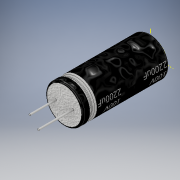
# Autodesk Inventor part: capacitor 2
Saved by Autodesk Inventor 2019 (Build 230136000, 136)
## iProperties
Created: 2019-08-10
Part Number: capacitor 2
Material: Типовые
Document SubType Name: Modeling
Designer: azizg
Density: 1 g/cm^3
Appearance: По умолчанию
Author: azizg
Autodesk Inventor part; units mm, degrees
sketch "Эскиз1" plane through (0, 0, 0) normal (0, 0, 1) x (1, 0, 0)
  line L0 (-13.3395, 0) -> (13.3395, 0)
  line L1 (0, 13.3395) -> (0, -13.3395)
  circle A0 centre (0, 0) radius 11
  dimension "d0" = 22
  constraints: 6 midpoint, 4 end point, 1 centre point, 1 coincident, 1 horizontal, 1 vertical
  measures "d0" diameter of A0
extrude "Выдавливание1" add sketch "Эскиз1" along normal mid plane 50
ref_plane "РабПлоскость3" through (0, 0, 20) normal (0, 0, 1) x (1, 0, 0)
sketch "Эскиз3" plane through (0, 0, 20) normal (0, 0, 1) x (1, 0, 0)
  line L0 (-22, 0) -> (25.1429, 0)
  line L1 (0, 25.1429) -> (0, -23.5714)
  circle A0 centre (0, 0) radius 11
  circle A1 centre (0, 0) radius 10
  dimension "d5" = 22
  dimension "d6" = 20
  constraints: 4 end point, 2 centre point, 2 coincident, 2 point on line, 1 horizontal, 1 vertical
  measures "d5" diameter of A0
  measures "d6" diameter of A1
extrude "Выдавливание2" cut sketch "Эскиз3" against normal blind 2 contours A1 L1 A0 L0 | L0 A0 L1 A1 | A1 L0 A0 L1 | L1 A0 L0 A1
fillet "Сопряжение1" radius 1 6 edges at (-11, 0, 20) (-11, 0, 18) (-10, 0, 18) (-10, 0, 20) (-11, 0, 25) (-11, 0, -25)
sketch "Эскиз4" plane through (0, 0, -25) normal (0, 0, -1) x (-1, 0, 0)
  line L0 (1.547, 4.223) -> (-2.9486, 4.223) construction
  line L1 (-2.9486, 4.223) -> (-2.9486, -4.5142) construction
  line L2 (-2.9486, -4.5142) -> (1.547, -4.5142) construction
  line L3 (1.547, -4.5142) -> (1.547, 4.223) construction
  line L4 (-1.1823, 0.0186) -> (-0.1499, 0.0186)
  line L5 (-0.1499, 0.0186) -> (-0.1499, 1.0511)
  line L6 (-0.1499, 1.0511) -> (0.191, 1.0511)
  line L7 (0.191, 1.0511) -> (0.191, 0.0186)
  line L8 (0.191, 0.0186) -> (1.2235, 0.0186)
  line L9 (1.2235, 0.0186) -> (1.2235, -0.3099)
  line L10 (1.2235, -0.3099) -> (0.191, -0.3099)
  line L11 (0.191, -0.3099) -> (0.191, -1.3423)
  line L12 (0.191, -1.3423) -> (-0.1499, -1.3423)
  line L13 (-0.1499, -1.3423) -> (-0.1499, -0.3099)
  line L14 (-0.1499, -0.3099) -> (-1.1823, -0.3099)
  line L15 (-1.1823, -0.3099) -> (-1.1823, 0.0186)
  point P0 (0, 0)
  dimension "d0" = 22
  constraints: 2 other
extrude "Выдавливание3" add sketch "Эскиз4" against normal blind 0.1
sketch "Эскиз5" plane through (0, 0, -25) normal (0, 0, -1) x (-1, 0, 0)
  line L0 (-1.5437, 1.0709) -> (1.5067, 1.0709) construction
  line L1 (1.5067, 1.0709) -> (1.5067, -1.3226) construction
  line L2 (1.5067, -1.3226) -> (-1.5437, -1.3226) construction
  line L3 (-1.5437, -1.3226) -> (-1.5437, 1.0709) construction
  line L4 (1.1856, -0.2901) -> (0.1532, -0.2901)
  line L5 (0.1532, -0.2901) -> (0.1532, -1.3226)
  line L6 (0.1532, -1.3226) -> (-0.1877, -1.3226)
  line L7 (-0.1877, -1.3226) -> (-0.1877, -0.2901)
  line L8 (-0.1877, -0.2901) -> (-1.2202, -0.2901)
  line L9 (-1.2202, -0.2901) -> (-1.2202, 0.0384)
  line L10 (-1.2202, 0.0384) -> (-0.1877, 0.0384)
  line L11 (-0.1877, 0.0384) -> (-0.1877, 1.0709)
  line L12 (-0.1877, 1.0709) -> (0.1532, 1.0709)
  line L13 (0.1532, 1.0709) -> (0.1532, 0.0384)
  line L14 (0.1532, 0.0384) -> (1.1856, 0.0384)
  line L15 (1.1856, 0.0384) -> (1.1856, -0.2901)
  point P0 (0, 0)
  dimension "d0" = 22
  constraints: 2 other
extrude "Выдавливание4" add sketch "Эскиз5" against normal blind 0.1
ref_plane "РабПлоскость4" through (11, 0, 0) normal (1, 0, 0) x (0, 1, 0)
sketch "Эскиз6" plane through (11, 0, 0) normal (1, 0, 0) x (0, 1, 0)
  line L0 (-4.859, -23.88) -> (-4.859, -8.4004) construction
  line L1 (-4.859, -8.4004) -> (3.8671, -8.4004) construction
  line L2 (3.8671, -8.4004) -> (3.8671, -23.88) construction
  line L3 (3.8671, -23.88) -> (-4.859, -23.88) construction
  line L4 (-5.3548, 2.6762) -> (-5.3548, 16.9441) construction
  line L5 (-5.3548, 16.9441) -> (3.3351, 16.9441) construction
  line L6 (3.3351, 16.9441) -> (3.3351, 2.6762) construction
  line L7 (3.3351, 2.6762) -> (-5.3548, 2.6762) construction
  line L8 (-1.7493, -21.9312) -> (-1.7493, -23.4181)
  line L9 (-1.7493, -23.4181) -> (-2.0605, -23.4181)
  line L10 (-2.0605, -23.4181) -> (-2.0605, -22.8648)
  line L11 (-2.0605, -22.8648) -> (-4.1032, -22.8648)
  line L12 (-4.1032, -22.8648) -> (-4.1032, -23.4181)
  line L13 (-4.1032, -23.4181) -> (-4.3823, -23.4181)
  spline S0 degree 2 poles (-4.3823, -23.4181) (-4.3823, -23.1044) (-4.5601, -22.808) (-4.8071, -22.7883) knots 0 0 0 1 2 2 2
  line L14 (-4.8071, -22.7883) -> (-4.8071, -22.4721)
  line L15 (-4.8071, -22.4721) -> (-2.0605, -22.4721)
  line L16 (-2.0605, -22.4721) -> (-2.0605, -21.9312)
  line L17 (-2.0605, -21.9312) -> (-1.7493, -21.9312)
  spline S1 degree 2 poles (-3.2733, -19.4735) (-2.4532, -19.4735) (-1.685, -19.9502) (-1.685, -20.4467) knots 0 0 0 1 2 2 2
  spline S2 degree 2 poles (-1.685, -20.4467) (-1.685, -20.9506) (-2.468, -21.4223) (-3.2708, -21.4223) knots 0 0 0 1 2 2 2
  spline S3 degree 2 poles (-3.2708, -21.4223) (-4.0958, -21.4223) (-4.859, -20.9456) (-4.859, -20.4467) knots 0 0 0 1 2 2 2
  spline S4 degree 2 poles (-4.859, -20.4467) (-4.859, -19.9453) (-4.0686, -19.4735) (-3.2733, -19.4735) knots 0 0 0 1 2 2 2
  spline S5 degree 2 poles (-2.3445, -19.9971) (-2.4952, -19.9379) (-2.9596, -19.8885) (-3.2733, -19.8885) knots 0 0 0 1 2 2 2
  spline S6 degree 2 poles (-3.2733, -19.8885) (-3.5869, -19.8885) (-4.0488, -19.9379) (-4.2044, -19.9996) knots 0 0 0 1 2 2 2
  spline S7 degree 2 poles (-4.2044, -19.9996) (-4.3601, -20.0614) (-4.5206, -20.2763) (-4.5206, -20.4467) knots 0 0 0 1 2 2 2
  spline S8 degree 2 poles (-4.5206, -20.4467) (-4.5206, -20.6171) (-4.3601, -20.8369) (-4.1995, -20.9012) knots 0 0 0 1 2 2 2
  spline S9 degree 2 poles (-4.1995, -20.9012) (-4.0439, -20.9629) (-3.5697, -21.0074) (-3.2708, -21.0074) knots 0 0 0 1 2 2 2
  spline S10 degree 2 poles (-3.2708, -21.0074) (-2.9497, -21.0074) (-2.5199, -20.9679) (-2.3519, -20.9036) knots 0 0 0 1 2 2 2
  spline S11 degree 2 poles (-2.3519, -20.9036) (-2.1939, -20.8444) (-2.0234, -20.6245) (-2.0234, -20.4467) knots 0 0 0 1 2 2 2
  spline S12 degree 2 poles (-2.0234, -20.4467) (-2.0234, -20.2787) (-2.184, -20.0589) (-2.3445, -19.9971) knots 0 0 0 1 2 2 2
  spline S13 degree 2 poles (-3.2733, -17.1863) (-2.4532, -17.1863) (-1.685, -17.663) (-1.685, -18.1594) knots 0 0 0 1 2 2 2
  spline S14 degree 2 poles (-1.685, -18.1594) (-1.685, -18.6633) (-2.468, -19.1351) (-3.2708, -19.1351) knots 0 0 0 1 2 2 2
  spline S15 degree 2 poles (-3.2708, -19.1351) (-4.0958, -19.1351) (-4.859, -18.6584) (-4.859, -18.1594) knots 0 0 0 1 2 2 2
  spline S16 degree 2 poles (-4.859, -18.1594) (-4.859, -17.658) (-4.0686, -17.1863) (-3.2733, -17.1863) knots 0 0 0 1 2 2 2
  spline S17 degree 2 poles (-2.3445, -17.7099) (-2.4952, -17.6506) (-2.9596, -17.6012) (-3.2733, -17.6012) knots 0 0 0 1 2 2 2
  spline S18 degree 2 poles (-3.2733, -17.6012) (-3.5869, -17.6012) (-4.0488, -17.6506) (-4.2044, -17.7124) knots 0 0 0 1 2 2 2
  spline S19 degree 2 poles (-4.2044, -17.7124) (-4.3601, -17.7741) (-4.5206, -17.989) (-4.5206, -18.1594) knots 0 0 0 1 2 2 2
  spline S20 degree 2 poles (-4.5206, -18.1594) (-4.5206, -18.3299) (-4.3601, -18.5497) (-4.1995, -18.6139) knots 0 0 0 1 2 2 2
  spline S21 degree 2 poles (-4.1995, -18.6139) (-4.0439, -18.6757) (-3.5697, -18.7201) (-3.2708, -18.7201) knots 0 0 0 1 2 2 2
  spline S22 degree 2 poles (-3.2708, -18.7201) (-2.9497, -18.7201) (-2.5199, -18.6806) (-2.3519, -18.6164) knots 0 0 0 1 2 2 2
  spline S23 degree 2 poles (-2.3519, -18.6164) (-2.1939, -18.5571) (-2.0234, -18.3373) (-2.0234, -18.1594) knots 0 0 0 1 2 2 2
  spline S24 degree 2 poles (-2.0234, -18.1594) (-2.0234, -17.9915) (-2.184, -17.7717) (-2.3445, -17.7099) knots 0 0 0 1 2 2 2
  line L18 (-4.7973, -14.4989) -> (-1.7493, -15.5486)
  line L19 (-1.7493, -15.5486) -> (-1.7493, -15.9858)
  line L20 (-1.7493, -15.9858) -> (-4.7973, -17.0356)
  line L21 (-4.7973, -17.0356) -> (-4.7973, -16.6009)
  line L22 (-4.7973, -16.6009) -> (-2.2655, -15.7561)
  line L23 (-2.2655, -15.7561) -> (-4.7973, -14.9114)
  line L24 (-4.7973, -14.9114) -> (-4.7973, -14.4989)
  line L25 (3.2692, -21.778) -> (3.2692, -23.6577)
  line L26 (3.2692, -23.6577) -> (2.8369, -23.6577)
  spline S25 degree 2 poles (2.8369, -23.6577) (2.6468, -23.4552) (2.2935, -23.0945) (2.1034, -22.9216) knots 0 0 0 1 2 2 2
  spline S26 degree 2 poles (2.1034, -22.9216) (1.7205, -22.5734) (1.2611, -22.319) (1.0165, -22.319) knots 0 0 0 1 2 2 2
  spline S27 degree 2 poles (1.0165, -22.319) (0.8881, -22.319) (0.6954, -22.398) (0.6337, -22.4696) knots 0 0 0 1 2 2 2
  spline S28 degree 2 poles (0.6337, -22.4696) (0.5719, -22.5413) (0.5102, -22.729) (0.5102, -22.8426) knots 0 0 0 1 2 2 2
  spline S29 degree 2 poles (0.5102, -22.8426) (0.5102, -22.9513) (0.5645, -23.1736) (0.6065, -23.2749) knots 0 0 0 1 2 2 2
  spline S30 degree 2 poles (0.6065, -23.2749) (0.6411, -23.3613) (0.7399, -23.5219) (0.7745, -23.5713) knots 0 0 0 1 2 2 2
  line L27 (0.7745, -23.5713) -> (0.7745, -23.5935)
  line L28 (0.7745, -23.5935) -> (0.3398, -23.5935)
  spline S31 degree 2 poles (0.3398, -23.5935) (0.278, -23.4675) (0.157, -23.0155) (0.157, -22.813) knots 0 0 0 1 2 2 2
  spline S32 degree 2 poles (0.157, -22.813) (0.157, -22.3856) (0.609, -21.904) (0.9943, -21.904) knots 0 0 0 1 2 2 2
  spline S33 degree 2 poles (0.9943, -21.904) (1.1746, -21.904) (1.476, -21.988) (1.6044, -22.0621) knots 0 0 0 1 2 2 2
  spline S34 degree 2 poles (1.6044, -22.0621) (1.7378, -22.1362) (1.9996, -22.3511) (2.1256, -22.4696) knots 0 0 0 1 2 2 2
  spline S35 degree 2 poles (2.1256, -22.4696) (2.3355, -22.6623) (2.7851, -23.1341) (2.916, -23.2749) knots 0 0 0 1 2 2 2
  line L29 (2.916, -23.2749) -> (2.916, -21.778)
  line L30 (2.916, -21.778) -> (3.2692, -21.778)
  line L31 (3.2692, -19.4908) -> (3.2692, -21.3705)
  line L32 (3.2692, -21.3705) -> (2.8369, -21.3705)
  spline S36 degree 2 poles (2.8369, -21.3705) (2.6468, -21.1679) (2.2935, -20.8073) (2.1034, -20.6344) knots 0 0 0 1 2 2 2
  spline S37 degree 2 poles (2.1034, -20.6344) (1.7205, -20.2861) (1.2611, -20.0317) (1.0165, -20.0317) knots 0 0 0 1 2 2 2
  spline S38 degree 2 poles (1.0165, -20.0317) (0.8881, -20.0317) (0.6954, -20.1108) (0.6337, -20.1824) knots 0 0 0 1 2 2 2
  spline S39 degree 2 poles (0.6337, -20.1824) (0.5719, -20.254) (0.5102, -20.4417) (0.5102, -20.5554) knots 0 0 0 1 2 2 2
  spline S40 degree 2 poles (0.5102, -20.5554) (0.5102, -20.664) (0.5645, -20.8863) (0.6065, -20.9876) knots 0 0 0 1 2 2 2
  spline S41 degree 2 poles (0.6065, -20.9876) (0.6411, -21.0741) (0.7399, -21.2346) (0.7745, -21.284) knots 0 0 0 1 2 2 2
  line L33 (0.7745, -21.284) -> (0.7745, -21.3063)
  line L34 (0.7745, -21.3063) -> (0.3398, -21.3063)
  spline S42 degree 2 poles (0.3398, -21.3063) (0.278, -21.1803) (0.157, -20.7283) (0.157, -20.5257) knots 0 0 0 1 2 2 2
  spline S43 degree 2 poles (0.157, -20.5257) (0.157, -20.0984) (0.609, -19.6168) (0.9943, -19.6168) knots 0 0 0 1 2 2 2
  spline S44 degree 2 poles (0.9943, -19.6168) (1.1746, -19.6168) (1.476, -19.7007) (1.6044, -19.7748) knots 0 0 0 1 2 2 2
  spline S45 degree 2 poles (1.6044, -19.7748) (1.7378, -19.8489) (1.9996, -20.0638) (2.1256, -20.1824) knots 0 0 0 1 2 2 2
  spline S46 degree 2 poles (2.1256, -20.1824) (2.3355, -20.3751) (2.7851, -20.8468) (2.916, -20.9876) knots 0 0 0 1 2 2 2
  line L35 (2.916, -20.9876) -> (2.916, -19.4908)
  line L36 (2.916, -19.4908) -> (3.2692, -19.4908)
  spline S47 degree 2 poles (1.7452, -17.1863) (2.5652, -17.1863) (3.3334, -17.663) (3.3334, -18.1594) knots 0 0 0 1 2 2 2
  spline S48 degree 2 poles (3.3334, -18.1594) (3.3334, -18.6633) (2.5504, -19.1351) (1.7477, -19.1351) knots 0 0 0 1 2 2 2
  spline S49 degree 2 poles (1.7477, -19.1351) (0.9227, -19.1351) (0.1595, -18.6584) (0.1595, -18.1594) knots 0 0 0 1 2 2 2
  spline S50 degree 2 poles (0.1595, -18.1594) (0.1595, -17.658) (0.9499, -17.1863) (1.7452, -17.1863) knots 0 0 0 1 2 2 2
  spline S51 degree 2 poles (2.6739, -17.7099) (2.5233, -17.6506) (2.0589, -17.6012) (1.7452, -17.6012) knots 0 0 0 1 2 2 2
  spline S52 degree 2 poles (1.7452, -17.6012) (1.4315, -17.6012) (0.9696, -17.6506) (0.814, -17.7124) knots 0 0 0 1 2 2 2
  spline S53 degree 2 poles (0.814, -17.7124) (0.6584, -17.7741) (0.4978, -17.989) (0.4978, -18.1594) knots 0 0 0 1 2 2 2
  spline S54 degree 2 poles (0.4978, -18.1594) (0.4978, -18.3299) (0.6584, -18.5497) (0.8189, -18.6139) knots 0 0 0 1 2 2 2
  spline S55 degree 2 poles (0.8189, -18.6139) (0.9746, -18.6757) (1.4488, -18.7201) (1.7477, -18.7201) knots 0 0 0 1 2 2 2
  spline S56 degree 2 poles (1.7477, -18.7201) (2.0688, -18.7201) (2.4986, -18.6806) (2.6665, -18.6164) knots 0 0 0 1 2 2 2
  spline S57 degree 2 poles (2.6665, -18.6164) (2.8246, -18.5571) (2.995, -18.3373) (2.995, -18.1594) knots 0 0 0 1 2 2 2
  spline S58 degree 2 poles (2.995, -18.1594) (2.995, -17.9915) (2.8345, -17.7717) (2.6739, -17.7099) knots 0 0 0 1 2 2 2
  spline S59 degree 2 poles (1.7452, -14.899) (2.5652, -14.899) (3.3334, -15.3757) (3.3334, -15.8722) knots 0 0 0 1 2 2 2
  spline S60 degree 2 poles (3.3334, -15.8722) (3.3334, -16.3761) (2.5504, -16.8479) (1.7477, -16.8479) knots 0 0 0 1 2 2 2
  spline S61 degree 2 poles (1.7477, -16.8479) (0.9227, -16.8479) (0.1595, -16.3712) (0.1595, -15.8722) knots 0 0 0 1 2 2 2
  spline S62 degree 2 poles (0.1595, -15.8722) (0.1595, -15.3708) (0.9499, -14.899) (1.7452, -14.899) knots 0 0 0 1 2 2 2
  spline S63 degree 2 poles (2.6739, -15.4227) (2.5233, -15.3634) (2.0589, -15.314) (1.7452, -15.314) knots 0 0 0 1 2 2 2
  spline S64 degree 2 poles (1.7452, -15.314) (1.4315, -15.314) (0.9696, -15.3634) (0.814, -15.4251) knots 0 0 0 1 2 2 2
  spline S65 degree 2 poles (0.814, -15.4251) (0.6584, -15.4869) (0.4978, -15.7018) (0.4978, -15.8722) knots 0 0 0 1 2 2 2
  spline S66 degree 2 poles (0.4978, -15.8722) (0.4978, -16.0426) (0.6584, -16.2625) (0.8189, -16.3267) knots 0 0 0 1 2 2 2
  spline S67 degree 2 poles (0.8189, -16.3267) (0.9746, -16.3884) (1.4488, -16.4329) (1.7477, -16.4329) knots 0 0 0 1 2 2 2
  spline S68 degree 2 poles (1.7477, -16.4329) (2.0688, -16.4329) (2.4986, -16.3934) (2.6665, -16.3292) knots 0 0 0 1 2 2 2
  spline S69 degree 2 poles (2.6665, -16.3292) (2.8246, -16.2699) (2.995, -16.0501) (2.995, -15.8722) knots 0 0 0 1 2 2 2
  spline S70 degree 2 poles (2.995, -15.8722) (2.995, -15.7043) (2.8345, -15.4844) (2.6739, -15.4227) knots 0 0 0 1 2 2 2
  line L37 (3.2692, -12.6735) -> (3.2692, -13.0589)
  line L38 (3.2692, -13.0589) -> (3.0173, -13.0589)
  spline S71 degree 2 poles (3.0173, -13.0589) (3.1729, -13.2367) (3.3334, -13.5553) (3.3334, -13.7529) knots 0 0 0 1 2 2 2
  spline S72 degree 2 poles (3.3334, -13.7529) (3.3334, -13.9011) (3.2346, -14.1654) (3.1284, -14.2618) knots 0 0 0 1 2 2 2
  spline S73 degree 2 poles (3.1284, -14.2618) (3.0222, -14.3606) (2.6986, -14.4692) (2.4664, -14.4692) knots 0 0 0 1 2 2 2
  line L39 (2.4664, -14.4692) -> (0.982, -14.4692)
  line L40 (0.982, -14.4692) -> (0.982, -14.0839)
  line L41 (0.982, -14.0839) -> (2.2861, -14.0839)
  spline S74 degree 2 poles (2.2861, -14.0839) (2.4689, -14.0839) (2.7085, -14.0568) (2.7974, -14.0098) knots 0 0 0 1 2 2 2
  spline S75 degree 2 poles (2.7974, -14.0098) (2.8863, -13.9629) (2.9679, -13.8023) (2.9679, -13.6517) knots 0 0 0 1 2 2 2
  spline S76 degree 2 poles (2.9679, -13.6517) (2.9679, -13.5109) (2.8073, -13.1922) (2.6912, -13.0589) knots 0 0 0 1 2 2 2
  line L42 (2.6912, -13.0589) -> (0.982, -13.0589)
  line L43 (0.982, -13.0589) -> (0.982, -12.6735)
  line L44 (0.982, -12.6735) -> (3.2692, -12.6735)
  line L45 (0.5818, -10.2628) -> (0.5818, -11.6806)
  line L46 (0.5818, -11.6806) -> (1.4414, -11.6806)
  line L47 (1.4414, -11.6806) -> (1.4414, -10.3221)
  line L48 (1.4414, -10.3221) -> (1.802, -10.3221)
  line L49 (1.802, -10.3221) -> (1.802, -11.6806)
  line L50 (1.802, -11.6806) -> (3.2692, -11.6806)
  line L51 (3.2692, -11.6806) -> (3.2692, -12.0857)
  line L52 (3.2692, -12.0857) -> (0.2212, -12.0857)
  line L53 (0.2212, -12.0857) -> (0.2212, -10.2628)
  line L54 (0.2212, -10.2628) -> (0.5818, -10.2628)
  line L55 (-2.245, 4.6251) -> (-2.245, 3.1381)
  line L56 (-2.245, 3.1381) -> (-2.5562, 3.1381)
  line L57 (-2.5562, 3.1381) -> (-2.5562, 3.6914)
  line L58 (-2.5562, 3.6914) -> (-4.5989, 3.6914)
  line L59 (-4.5989, 3.6914) -> (-4.5989, 3.1381)
  line L60 (-4.5989, 3.1381) -> (-4.878, 3.1381)
  spline S77 degree 2 poles (-4.878, 3.1381) (-4.878, 3.4518) (-5.0559, 3.7482) (-5.3029, 3.768) knots 0 0 0 1 2 2 2
  line L61 (-5.3029, 3.768) -> (-5.3029, 4.0841)
  line L62 (-5.3029, 4.0841) -> (-2.5562, 4.0841)
  line L63 (-2.5562, 4.0841) -> (-2.5562, 4.6251)
  line L64 (-2.5562, 4.6251) -> (-2.245, 4.6251)
  spline S78 degree 2 poles (-3.769, 7.0827) (-2.949, 7.0827) (-2.1808, 6.606) (-2.1808, 6.1095) knots 0 0 0 1 2 2 2
  spline S79 degree 2 poles (-2.1808, 6.1095) (-2.1808, 5.6057) (-2.9638, 5.1339) (-3.7665, 5.1339) knots 0 0 0 1 2 2 2
  spline S80 degree 2 poles (-3.7665, 5.1339) (-4.5915, 5.1339) (-5.3548, 5.6106) (-5.3548, 6.1095) knots 0 0 0 1 2 2 2
  spline S81 degree 2 poles (-5.3548, 6.1095) (-5.3548, 6.611) (-4.5643, 7.0827) (-3.769, 7.0827) knots 0 0 0 1 2 2 2
  spline S82 degree 2 poles (-2.8403, 6.5591) (-2.9909, 6.6184) (-3.4553, 6.6678) (-3.769, 6.6678) knots 0 0 0 1 2 2 2
  spline S83 degree 2 poles (-3.769, 6.6678) (-4.0827, 6.6678) (-4.5446, 6.6184) (-4.7002, 6.5566) knots 0 0 0 1 2 2 2
  spline S84 degree 2 poles (-4.7002, 6.5566) (-4.8558, 6.4949) (-5.0164, 6.28) (-5.0164, 6.1095) knots 0 0 0 1 2 2 2
  spline S85 degree 2 poles (-5.0164, 6.1095) (-5.0164, 5.9391) (-4.8558, 5.7193) (-4.6953, 5.6551) knots 0 0 0 1 2 2 2
  spline S86 degree 2 poles (-4.6953, 5.6551) (-4.5396, 5.5933) (-4.0654, 5.5488) (-3.7665, 5.5488) knots 0 0 0 1 2 2 2
  spline S87 degree 2 poles (-3.7665, 5.5488) (-3.4454, 5.5488) (-3.0156, 5.5884) (-2.8477, 5.6526) knots 0 0 0 1 2 2 2
  spline S88 degree 2 poles (-2.8477, 5.6526) (-2.6896, 5.7119) (-2.5192, 5.9317) (-2.5192, 6.1095) knots 0 0 0 1 2 2 2
  spline S89 degree 2 poles (-2.5192, 6.1095) (-2.5192, 6.2775) (-2.6797, 6.4973) (-2.8403, 6.5591) knots 0 0 0 1 2 2 2
  spline S90 degree 2 poles (-3.769, 9.37) (-2.949, 9.37) (-2.1808, 8.8932) (-2.1808, 8.3968) knots 0 0 0 1 2 2 2
  spline S91 degree 2 poles (-2.1808, 8.3968) (-2.1808, 7.8929) (-2.9638, 7.4211) (-3.7665, 7.4211) knots 0 0 0 1 2 2 2
  spline S92 degree 2 poles (-3.7665, 7.4211) (-4.5915, 7.4211) (-5.3548, 7.8978) (-5.3548, 8.3968) knots 0 0 0 1 2 2 2
  spline S93 degree 2 poles (-5.3548, 8.3968) (-5.3548, 8.8982) (-4.5643, 9.37) (-3.769, 9.37) knots 0 0 0 1 2 2 2
  spline S94 degree 2 poles (-2.8403, 8.8463) (-2.9909, 8.9056) (-3.4553, 8.955) (-3.769, 8.955) knots 0 0 0 1 2 2 2
  spline S95 degree 2 poles (-3.769, 8.955) (-4.0827, 8.955) (-4.5446, 8.9056) (-4.7002, 8.8438) knots 0 0 0 1 2 2 2
  spline S96 degree 2 poles (-4.7002, 8.8438) (-4.8558, 8.7821) (-5.0164, 8.5672) (-5.0164, 8.3968) knots 0 0 0 1 2 2 2
  spline S97 degree 2 poles (-5.0164, 8.3968) (-5.0164, 8.2263) (-4.8558, 8.0065) (-4.6953, 7.9423) knots 0 0 0 1 2 2 2
  spline S98 degree 2 poles (-4.6953, 7.9423) (-4.5396, 7.8805) (-4.0654, 7.8361) (-3.7665, 7.8361) knots 0 0 0 1 2 2 2
  spline S99 degree 2 poles (-3.7665, 7.8361) (-3.4454, 7.8361) (-3.0156, 7.8756) (-2.8477, 7.9398) knots 0 0 0 1 2 2 2
  spline S100 degree 2 poles (-2.8477, 7.9398) (-2.6896, 7.9991) (-2.5192, 8.2189) (-2.5192, 8.3968) knots 0 0 0 1 2 2 2
  spline S101 degree 2 poles (-2.5192, 8.3968) (-2.5192, 8.5647) (-2.6797, 8.7846) (-2.8403, 8.8463) knots 0 0 0 1 2 2 2
  line L65 (-5.293, 12.0573) -> (-2.245, 11.0076)
  line L66 (-2.245, 11.0076) -> (-2.245, 10.5704)
  line L67 (-2.245, 10.5704) -> (-5.293, 9.5206)
  line L68 (-5.293, 9.5206) -> (-5.293, 9.9554)
  line L69 (-5.293, 9.9554) -> (-2.7612, 10.8001)
  line L70 (-2.7612, 10.8001) -> (-5.293, 11.6448)
  line L71 (-5.293, 11.6448) -> (-5.293, 12.0573)
  line L72 (2.7735, 4.7782) -> (2.7735, 2.8985)
  line L73 (2.7735, 2.8985) -> (2.3412, 2.8985)
  spline S102 degree 2 poles (2.3412, 2.8985) (2.151, 3.1011) (1.7978, 3.4617) (1.6076, 3.6346) knots 0 0 0 1 2 2 2
  spline S103 degree 2 poles (1.6076, 3.6346) (1.2248, 3.9829) (0.7653, 4.2373) (0.5208, 4.2373) knots 0 0 0 1 2 2 2
  spline S104 degree 2 poles (0.5208, 4.2373) (0.3924, 4.2373) (0.1997, 4.1582) (0.1379, 4.0866) knots 0 0 0 1 2 2 2
  spline S105 degree 2 poles (0.1379, 4.0866) (0.0762, 4.015) (0.0144, 3.8272) (0.0144, 3.7136) knots 0 0 0 1 2 2 2
  spline S106 degree 2 poles (0.0144, 3.7136) (0.0144, 3.6049) (0.0688, 3.3826) (0.1108, 3.2814) knots 0 0 0 1 2 2 2
  spline S107 degree 2 poles (0.1108, 3.2814) (0.1454, 3.1949) (0.2442, 3.0344) (0.2787, 2.985) knots 0 0 0 1 2 2 2
  line L74 (0.2787, 2.985) -> (0.2787, 2.9627)
  line L75 (0.2787, 2.9627) -> (-0.156, 2.9627)
  spline S108 degree 2 poles (-0.156, 2.9627) (-0.2177, 3.0887) (-0.3388, 3.5407) (-0.3388, 3.7433) knots 0 0 0 1 2 2 2
  spline S109 degree 2 poles (-0.3388, 3.7433) (-0.3388, 4.1706) (0.1132, 4.6522) (0.4986, 4.6522) knots 0 0 0 1 2 2 2
  spline S110 degree 2 poles (0.4986, 4.6522) (0.6789, 4.6522) (0.9802, 4.5682) (1.1087, 4.4941) knots 0 0 0 1 2 2 2
  spline S111 degree 2 poles (1.1087, 4.4941) (1.242, 4.42) (1.5039, 4.2052) (1.6298, 4.0866) knots 0 0 0 1 2 2 2
  spline S112 degree 2 poles (1.6298, 4.0866) (1.8398, 3.8939) (2.2893, 3.4222) (2.4202, 3.2814) knots 0 0 0 1 2 2 2
  line L76 (2.4202, 3.2814) -> (2.4202, 4.7782)
  line L77 (2.4202, 4.7782) -> (2.7735, 4.7782)
  line L78 (2.7735, 7.0654) -> (2.7735, 5.1858)
  line L79 (2.7735, 5.1858) -> (2.3412, 5.1858)
  spline S113 degree 2 poles (2.3412, 5.1858) (2.151, 5.3883) (1.7978, 5.7489) (1.6076, 5.9218) knots 0 0 0 1 2 2 2
  spline S114 degree 2 poles (1.6076, 5.9218) (1.2248, 6.2701) (0.7653, 6.5245) (0.5208, 6.5245) knots 0 0 0 1 2 2 2
  spline S115 degree 2 poles (0.5208, 6.5245) (0.3924, 6.5245) (0.1997, 6.4455) (0.1379, 6.3738) knots 0 0 0 1 2 2 2
  spline S116 degree 2 poles (0.1379, 6.3738) (0.0762, 6.3022) (0.0144, 6.1145) (0.0144, 6.0009) knots 0 0 0 1 2 2 2
  spline S117 degree 2 poles (0.0144, 6.0009) (0.0144, 5.8922) (0.0688, 5.6699) (0.1108, 5.5686) knots 0 0 0 1 2 2 2
  spline S118 degree 2 poles (0.1108, 5.5686) (0.1454, 5.4822) (0.2442, 5.3216) (0.2787, 5.2722) knots 0 0 0 1 2 2 2
  line L80 (0.2787, 5.2722) -> (0.2787, 5.25)
  line L81 (0.2787, 5.25) -> (-0.156, 5.25)
  spline S119 degree 2 poles (-0.156, 5.25) (-0.2177, 5.3759) (-0.3388, 5.828) (-0.3388, 6.0305) knots 0 0 0 1 2 2 2
  spline S120 degree 2 poles (-0.3388, 6.0305) (-0.3388, 6.4578) (0.1132, 6.9395) (0.4986, 6.9395) knots 0 0 0 1 2 2 2
  spline S121 degree 2 poles (0.4986, 6.9395) (0.6789, 6.9395) (0.9802, 6.8555) (1.1087, 6.7814) knots 0 0 0 1 2 2 2
  spline S122 degree 2 poles (1.1087, 6.7814) (1.242, 6.7073) (1.5039, 6.4924) (1.6298, 6.3738) knots 0 0 0 1 2 2 2
  spline S123 degree 2 poles (1.6298, 6.3738) (1.8398, 6.1812) (2.2893, 5.7094) (2.4202, 5.5686) knots 0 0 0 1 2 2 2
  line L82 (2.4202, 5.5686) -> (2.4202, 7.0654)
  line L83 (2.4202, 7.0654) -> (2.7735, 7.0654)
  spline S124 degree 2 poles (1.2495, 9.37) (2.0695, 9.37) (2.8377, 8.8932) (2.8377, 8.3968) knots 0 0 0 1 2 2 2
  spline S125 degree 2 poles (2.8377, 8.3968) (2.8377, 7.8929) (2.0547, 7.4211) (1.2519, 7.4211) knots 0 0 0 1 2 2 2
  spline S126 degree 2 poles (1.2519, 7.4211) (0.4269, 7.4211) (-0.3363, 7.8978) (-0.3363, 8.3968) knots 0 0 0 1 2 2 2
  spline S127 degree 2 poles (-0.3363, 8.3968) (-0.3363, 8.8982) (0.4541, 9.37) (1.2495, 9.37) knots 0 0 0 1 2 2 2
  spline S128 degree 2 poles (2.1782, 8.8463) (2.0275, 8.9056) (1.5631, 8.955) (1.2495, 8.955) knots 0 0 0 1 2 2 2
  spline S129 degree 2 poles (1.2495, 8.955) (0.9358, 8.955) (0.4739, 8.9056) (0.3183, 8.8438) knots 0 0 0 1 2 2 2
  spline S130 degree 2 poles (0.3183, 8.8438) (0.1626, 8.7821) (0.0021, 8.5672) (0.0021, 8.3968) knots 0 0 0 1 2 2 2
  spline S131 degree 2 poles (0.0021, 8.3968) (0.0021, 8.2263) (0.1626, 8.0065) (0.3232, 7.9423) knots 0 0 0 1 2 2 2
  spline S132 degree 2 poles (0.3232, 7.9423) (0.4788, 7.8805) (0.953, 7.8361) (1.2519, 7.8361) knots 0 0 0 1 2 2 2
  spline S133 degree 2 poles (1.2519, 7.8361) (1.573, 7.8361) (2.0028, 7.8756) (2.1708, 7.9398) knots 0 0 0 1 2 2 2
  spline S134 degree 2 poles (2.1708, 7.9398) (2.3288, 7.9991) (2.4993, 8.2189) (2.4993, 8.3968) knots 0 0 0 1 2 2 2
  spline S135 degree 2 poles (2.4993, 8.3968) (2.4993, 8.5647) (2.3387, 8.7846) (2.1782, 8.8463) knots 0 0 0 1 2 2 2
  spline S136 degree 2 poles (1.2495, 11.6572) (2.0695, 11.6572) (2.8377, 11.1805) (2.8377, 10.684) knots 0 0 0 1 2 2 2
  spline S137 degree 2 poles (2.8377, 10.684) (2.8377, 10.1801) (2.0547, 9.7084) (1.2519, 9.7084) knots 0 0 0 1 2 2 2
  spline S138 degree 2 poles (1.2519, 9.7084) (0.4269, 9.7084) (-0.3363, 10.1851) (-0.3363, 10.684) knots 0 0 0 1 2 2 2
  spline S139 degree 2 poles (-0.3363, 10.684) (-0.3363, 11.1854) (0.4541, 11.6572) (1.2495, 11.6572) knots 0 0 0 1 2 2 2
  spline S140 degree 2 poles (2.1782, 11.1336) (2.0275, 11.1928) (1.5631, 11.2422) (1.2495, 11.2422) knots 0 0 0 1 2 2 2
  spline S141 degree 2 poles (1.2495, 11.2422) (0.9358, 11.2422) (0.4739, 11.1928) (0.3183, 11.1311) knots 0 0 0 1 2 2 2
  spline S142 degree 2 poles (0.3183, 11.1311) (0.1626, 11.0693) (0.0021, 10.8544) (0.0021, 10.684) knots 0 0 0 1 2 2 2
  spline S143 degree 2 poles (0.0021, 10.684) (0.0021, 10.5136) (0.1626, 10.2937) (0.3232, 10.2295) knots 0 0 0 1 2 2 2
  spline S144 degree 2 poles (0.3232, 10.2295) (0.4788, 10.1678) (0.953, 10.1233) (1.2519, 10.1233) knots 0 0 0 1 2 2 2
  spline S145 degree 2 poles (1.2519, 10.1233) (1.573, 10.1233) (2.0028, 10.1628) (2.1708, 10.2271) knots 0 0 0 1 2 2 2
  spline S146 degree 2 poles (2.1708, 10.2271) (2.3288, 10.2863) (2.4993, 10.5062) (2.4993, 10.684) knots 0 0 0 1 2 2 2
  spline S147 degree 2 poles (2.4993, 10.684) (2.4993, 10.852) (2.3387, 11.0718) (2.1782, 11.1336) knots 0 0 0 1 2 2 2
  line L84 (2.7735, 13.8827) -> (2.7735, 13.4974)
  line L85 (2.7735, 13.4974) -> (2.5215, 13.4974)
  spline S148 degree 2 poles (2.5215, 13.4974) (2.6771, 13.3195) (2.8377, 13.0009) (2.8377, 12.8033) knots 0 0 0 1 2 2 2
  spline S149 degree 2 poles (2.8377, 12.8033) (2.8377, 12.6551) (2.7389, 12.3908) (2.6327, 12.2945) knots 0 0 0 1 2 2 2
  spline S150 degree 2 poles (2.6327, 12.2945) (2.5264, 12.1957) (2.2029, 12.087) (1.9707, 12.087) knots 0 0 0 1 2 2 2
  line L86 (1.9707, 12.087) -> (0.4862, 12.087)
  line L87 (0.4862, 12.087) -> (0.4862, 12.4723)
  line L88 (0.4862, 12.4723) -> (1.7904, 12.4723)
  spline S151 degree 2 poles (1.7904, 12.4723) (1.9732, 12.4723) (2.2128, 12.4995) (2.3017, 12.5464) knots 0 0 0 1 2 2 2
  spline S152 degree 2 poles (2.3017, 12.5464) (2.3906, 12.5933) (2.4721, 12.7539) (2.4721, 12.9046) knots 0 0 0 1 2 2 2
  spline S153 degree 2 poles (2.4721, 12.9046) (2.4721, 13.0453) (2.3116, 13.364) (2.1955, 13.4974) knots 0 0 0 1 2 2 2
  line L89 (2.1955, 13.4974) -> (0.4862, 13.4974)
  line L90 (0.4862, 13.4974) -> (0.4862, 13.8827)
  line L91 (0.4862, 13.8827) -> (2.7735, 13.8827)
  line L92 (0.0861, 16.2934) -> (0.0861, 14.8756)
  line L93 (0.0861, 14.8756) -> (0.9456, 14.8756)
  line L94 (0.9456, 14.8756) -> (0.9456, 16.2341)
  line L95 (0.9456, 16.2341) -> (1.3063, 16.2341)
  line L96 (1.3063, 16.2341) -> (1.3063, 14.8756)
  line L97 (1.3063, 14.8756) -> (2.7735, 14.8756)
  line L98 (2.7735, 14.8756) -> (2.7735, 14.4705)
  line L99 (2.7735, 14.4705) -> (-0.2745, 14.4705)
  line L100 (-0.2745, 14.4705) -> (-0.2745, 16.2934)
  line L101 (-0.2745, 16.2934) -> (0.0861, 16.2934)
  point P0 (0, 0)
  dimension "d0" = 22
  constraints: 4 other
extrude "Выдавливание5" cut sketch "Эскиз6" against normal blind 1.5
sketch "Эскиз7" plane through (0, 0, -25) normal (0, 0, -1) x (-1, 0, 0)
  line L0 (-4.6026, 5.6685) -> (4.6067, 5.6685) construction
  line L1 (4.6067, 5.6685) -> (4.6067, -5.9388) construction
  line L2 (4.6067, -5.9388) -> (-4.6026, -5.9388) construction
  line L3 (-4.6026, -5.9388) -> (-4.6026, 5.6685) construction
  line L4 (13.3395, 0) -> (-13.3395, 0) projected
  line L5 (0, 13.3395) -> (0, -13.3395) projected
  circle A0 centre (0, 0) radius 10 projected
  line L6 (1.2062, -0.2994) -> (0.1737, -0.2994)
  line L7 (0.1737, -0.2994) -> (0.1737, -1.3319)
  line L8 (0.1737, -1.3319) -> (-0.1672, -1.3319)
  line L9 (-0.1672, -1.3319) -> (-0.1672, -0.2994)
  line L10 (-0.1672, -0.2994) -> (-1.1996, -0.2994)
  line L11 (-1.1996, -0.2994) -> (-1.1996, 0.0291)
  line L12 (-1.1996, 0.0291) -> (-0.1672, 0.0291)
  line L13 (-0.1672, 0.0291) -> (-0.1672, 1.0616)
  line L14 (-0.1672, 1.0616) -> (0.1737, 1.0616)
  line L15 (0.1737, 1.0616) -> (0.1737, 0.0291)
  line L16 (0.1737, 0.0291) -> (1.2062, 0.0291)
  line L17 (1.2062, 0.0291) -> (1.2062, -0.2994)
  dimension "d0" = 22
  constraints: 2 other
extrude "Выдавливание6" cut sketch "Эскиз7" against normal blind 1.5 contours L17 L6 L7 L8 L5 L4 | L4 L5 L14 L15 L16 L17 | L5 L8 L9 L10 L11 L4 | L4 L11 L12 L13 L14 L5
ref_plane "РабПлоскость7" through (0, 0, 25) normal (0, 0, 1) x (1, 0, 0)
sketch "Эскиз9" plane through (0, 0, 25) normal (0, 0, 1) x (1, 0, 0)
  circle A0 centre (5, 0.0291) radius 0.5
  circle A1 centre (-5, 0) radius 0.5
  point P0 (0, 0)
  point P1 (-1.2062, 0.0291)
  dimension "d32" = 1
  dimension "d33" = 5
  dimension "d35" = 1
  dimension "d36" = 5
  constraints: 2 centre point
  measures "d32" diameter of A0
  measures "d33" horizontal distance of A0.centre point (0, 0)
  measures "d35" diameter of A1
  measures "d36" distance of A1.centre point (0, 0)
extrude "Выдавливание9" add sketch "Эскиз9" along normal blind 15
sketch "Эскиз10" plane through (5, 0.0291, 40) normal (0, 0, 1) x (1, 0, 0)
  circle A0 centre (0, 0) radius 0.5
  point P0 (-5, -0.0291)
  constraints: 1 centre point
extrude "Выдавливание10" add sketch "Эскиз10" along normal blind 5
